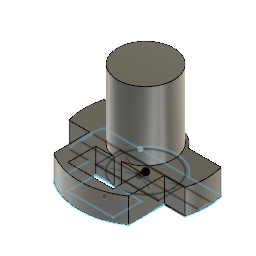
transmitter bracket (Autodesk Fusion 360 design; units mm, degrees)
Autodesk Fusion 360 part; units mm, degrees
sketch "Sketch1" plane through (0, 0, 0) normal (0, 0, 1) x (1, 0, 0)
  circle A0 centre (0, 0) radius 4.5
  line L0 (3.7508, -8.9624) -> (-3.5492, -8.9624)
  line L1 (-3.5492, -8.9624) -> (-3.5492, -4.4624)
  line L2 (-3.5492, -4.4624) -> (3.7508, -4.4624)
  line L3 (3.7508, -4.4624) -> (3.7508, -8.9624)
  line L4 (3.7508, -8.9624) -> (-3.5492, -4.4624) construction
  line L5 (-3.5492, -8.9624) -> (3.7508, -4.4624) construction
  line L6 (9.5, -1) -> (-9.5, -1)
  line L7 (-9.5, -1) -> (-9.5, 1)
  line L8 (-9.5, 1) -> (9.5, 1)
  line L9 (9.5, 1) -> (9.5, -1)
  line L10 (9.5, -1) -> (-9.5, 1) construction
  line L11 (-9.5, -1) -> (9.5, 1) construction
  line L12 (5, -3) -> (-5, -3)
  line L13 (-5, -3) -> (-5, 1)
  line L14 (-5, 1) -> (5, 1)
  line L15 (5, 1) -> (5, -3)
  line L16 (5, -3) -> (-5, 1) construction
  line L17 (-5, -3) -> (5, 1) construction
  arc A1 (-9.411, 2.7195) -> (-9.3254, -3) centre (0, 0) ccw
  arc A2 (-6.0086, -8.7611) -> (6.0086, -8.7611) centre (0, 0) ccw
  arc A3 (9.3254, -3) -> (9.411, 2.7195) centre (0, 0) ccw
  line L18 (-6.0086, -8.7611) -> (-6.0086, -3)
  line L19 (6.0086, -3) -> (6.0086, -8.7611)
  line L20 (-9.3254, -3) -> (-6.0086, -3)
  line L21 (-5, -3) -> (5, -3)
  line L22 (6.0086, -3) -> (9.3254, -3)
  line L23 (-9.411, 2.7195) -> (-4.1363, 2.7195)
  line L24 (-3.5853, 2.7195) -> (3.5853, 2.7195)
  line L25 (4.1363, 2.7195) -> (9.411, 2.7195)
  arc A4 (4.1363, 2.7195) -> (-4.1363, 2.7195) centre (0, 0) ccw
  point P0 (0.1008, -6.7124)
  point P1 (0, -1)
  dimension "d1" = 9
  dimension "d2" = 7.3
  dimension "d3" = 4.5
  dimension "d9" = 2
  dimension "d10" = 10
  dimension "d11" = 4
  constraint coincident A0.centre A1.centre
  constraint horizontal L0
  constraint perpendicular L0 L1
  constraint parallel L0 L2
  constraint parallel L1 L3
  constraint coincident L4 P0
  constraint coincident L5 P0
  constraint concentric A0 A1
  constraint horizontal L6
  constraint perpendicular L6 L7
  constraint parallel L6 L8
  constraint parallel L7 L9
  constraint coincident L10 A0.centre
  constraint coincident L11 A0.centre
  constraint horizontal L12
  constraint perpendicular L12 L13
  constraint parallel L12 L14
  constraint parallel L13 L15
  constraint coincident L16 P1
  constraint coincident L17 P1
  constraint midpoint L6 P1
  constraint horizontal L23
  constraint horizontal L20
  constraint concentric A1 A2
  constraint concentric A2 A3
  constraint coincident L19.start L20
  constraint collinear L20 L21
  constraint collinear L21 L22
  constraint coincident A0 L24.start
  constraint collinear L23 L24
  constraint coincident A0 L24.end
  constraint collinear L24 L25
  measures "d1" diameter of A0
  measures "d2" distance of L1.end L2.end
  measures "d3" distance of L0.end L1.end
  measures "d9" distance of L6.end L7.end
  measures "d10" distance of L13.end L14.end
  measures "d11" distance of L12.end L13.end
extrude "Extrude1" add sketch "Sketch1" along normal blind 4 contours A0 L24 | A0 L8 L14 L24 | A0 L6 L8 L14 L15 | A0 L6 L8 L14 | A0 L6 L8 L13 L14 | L6 L8 L9 L15 | A0 L6 L12 L21 | A0 L6 L12 L13 L21 | L6 L7 L8 L13 | A0 L6 L12 L15 L21 | A0 L2 L12 L21 | A1 A2 A3 L18 L19 L20 L22 L23 L25 A4
extrude "Extrude2" add sketch "Sketch1" along normal blind 15 contours A0 L24 | A0 L8 L14 L24 | A0 L6 L8 L14 | A0 L6 L12 L21 | A0 L2 L12 L21 | A0 L2
extrude "Extrude3" cut sketch "Sketch1" along normal blind 3 contours A0 L6 L8 L14 L15 | A0 L6 L8 L14 | A0 L6 L8 L13 L14 | L6 L8 L9 L15 | A0 L6 L12 L21 | A0 L6 L12 L13 L21 | L6 L7 L8 L13 | A0 L6 L12 L15 L21
